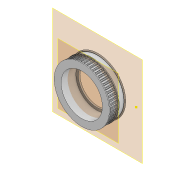
# Autodesk Inventor part: 20_Cube_Insert_rotational_filtermount_v3
Saved by Autodesk Inventor 2022 (Build 260153000, 153)
## iProperties
Created: 2022-02-14
Part Number: 20_Cube_Insert_rotational_filtermount_v3
Material: Generisch
Document SubType Name: Modeling
Designer: diederichbenedict
Density: 1 g/cm^3
Appearance: Vorgabe
Author: diederichbenedict
Autodesk Inventor part; units mm, degrees
ref_plane "YZ Plane" through (0, 0, 0) normal (1, 0, 0) x (0, 1, 0)
ref_plane "XZ Plane" through (0, 0, 0) normal (0, 1, 0) x (-1, 0, 0)
ref_plane "XY Plane" through (0, 0, 0) normal (0, 0, 1) x (1, 0, 0)
ref_plane "Arbeitsebene1" through (0, 0, 0) normal (0, 0, 1) x (1, 0, 0)
sketch "Skizze1" plane through (0, 0, 0) normal (0, 0, 1) x (1, 0, 0)
  circle A0 centre (-23.0919, -0.0207) radius 10 construction
  circle A1 centre (-5.7714, -10.0207) radius 3 construction
  circle A2 centre (-40.4124, -10.0207) radius 3 construction
  circle A3 centre (-23.0919, 19.9793) radius 3 construction
  circle A4 centre (-23.0919, -0.0207) radius 10 construction
  line L0 (1.8288, -17) -> (1.8288, 17) construction
  line L1 (1.8288, 17) -> (-1.746, 17) construction
  line L2 (-1.746, 17) -> (-6.0712, 21.3252) construction
  line L3 (-6.0712, 21.3252) -> (-6.0712, 24.9) construction
  line L4 (-6.0712, 24.9) -> (-40.0712, 24.9) construction
  line L5 (-40.0712, 24.9) -> (-40.0712, 21.3252) construction
  line L6 (-40.0712, 21.3252) -> (-44.3964, 17) construction
  line L7 (-44.3964, 17) -> (-47.9712, 17) construction
  line L8 (-47.9712, 17) -> (-47.9712, -17) construction
  line L9 (-44.3964, -17) -> (-47.9712, -17) construction
  line L10 (-40.0712, -21.3252) -> (-44.3964, -17) construction
  line L11 (-40.0712, -24.9) -> (-40.0712, -21.3252) construction
  line L12 (-6.1126, -24.9) -> (-40.0712, -24.9) construction
  line L13 (-6.1126, -24.9) -> (-6.1126, -21.3666) construction
  line L14 (-6.1126, -21.3666) -> (-1.746, -17) construction
  line L15 (-1.746, -17) -> (1.8288, -17) construction
  circle A5 centre (-23.0919, 19.9793) radius 2.5 construction
  circle A6 centre (-40.4124, -10.0207) radius 2.5 construction
  circle A7 centre (-5.7714, -10.0207) radius 2.5 construction
  circle A8 centre (-23.0919, -0.0207) radius 16.1
  circle A9 centre (-23.0919, 19.9793) radius 4 construction
  circle A10 centre (-5.7714, -10.0207) radius 4 construction
  circle A11 centre (-40.4124, -10.0207) radius 4 construction
  circle A12 centre (-23.0919, -0.0207) radius 12.575
  point P0 (0, 0)
  dimension "d4" = 8
  dimension "d5" = 8
  dimension "d6" = 8
  dimension "d7" = 32.2
  dimension "d8" = 25.15
  constraints: 5 centre point, 4 coincident
  measures "d4" diameter of A9
  measures "d5" diameter of A10
  measures "d6" diameter of A11
  measures "d7" diameter of A8
  measures "d8" diameter of A12
extrude "Extrusion1" add sketch "Skizze1" along normal blind 9
sketch "Skizze2" plane through (-23.0919, -0.0207, 9) normal (0, 0, 1) x (1, 0, 0)
  circle A0 centre (0, 0) radius 16.1 projected
  circle A1 centre (0, 0) radius 12.575 projected
  line L0 (16.6, 0.4) -> (15.6, 0.4)
  line L1 (15.6, 0.4) -> (15.6, -0.4)
  line L2 (15.6, -0.4) -> (16.6, -0.4)
  line L3 (16.6, -0.4) -> (16.6, 0.4)
  circle A2 centre (0, 0) radius 16.1 projected
  line L4 (16.6, 0.4) -> (15.6, -0.4) construction
  line L5 (15.6, 0.4) -> (16.6, -0.4) construction
  point P0 (23.0919, 0.0207)
  point P1 (16.1, 0)
  dimension "d9" = 1
  dimension "d10" = 0.8
  constraints: 12 end point, 2 midpoint, 2 parallel, 1 horizontal, 1 horizontal alignment, 1 perpendicular, 1 other
  measures "d9" distance of L2.end L1.end
  measures "d10" distance of L1.end L0.end
extrude "Extrusion2" add sketch "Skizze2" against normal blind 5 contours A0 L2 L1 L0 | A0 L0 L3 L2 picked at (15.7667, 0)
fillet "Rundung1" radius 0.2 4 edges at (-6.4919, -0.4207, 6.5) (-6.9969, -0.4207, 6.5) (-6.4919, 0.3793, 6.5) (-6.9969, 0.3793, 6.5)
pattern_circular "Runde Anordnung1" count 52 over 360 about axis through (-23.0919, -0.0207, 0) along (0, 0, 1) of "Rundung1", "Extrusion2"
sketch "Skizze3" plane through (0, 0, 9) normal (0, 0, 1) x (1, 0, 0)
  circle A0 centre (-23.0919, -0.0207) radius 12.575 projected
  circle A1 centre (-23.0919, -0.0207) radius 16.7976
  point P0 (0, 0)
  constraints: 1 centre point
extrude "Extrusion3" add sketch "Skizze3" along normal blind 0.5
ref_plane "Arbeitsebene2" through (-23.0919, -0.0207, 5.5) normal (0, 0, 1) x (1, 0, 0)
sketch "Skizze4" plane through (-23.0919, -0.0207, 4) normal (0, 0, 1) x (1, 0, 0)
  circle A0 centre (0, 0) radius 16.7976 projected
  circle A1 centre (0, 0) radius 12.575 projected
  point P0 (23.0919, 0.0207)
extrude "Extrusion4" add sketch "Skizze4" against normal blind 0.5
sketch "Skizze5" plane through (-23.0919, -0.0207, 0) normal (0, 0, -1) x (-1, 0, 0)
  circle A0 centre (0, 0) radius 16.7976 projected
  circle A1 centre (0, 0) radius 12.575 projected
  point P0 (-23.0919, 0.0207)
extrude "Extrusion5" add sketch "Skizze5" along normal blind 0.5
sketch "Skizze6" plane through (-23.0919, -0.0207, -0.5) normal (0, 0, -1) x (-1, 0, 0)
  point P0 (-23.0919, 0.0207)
sketch "Skizze7" plane through (-23.0919, -0.0207, -0.5) normal (0, 0, 1) x (1, 0, 0)
  circle A0 centre (0, 0) radius 12.575 projected
  circle A1 centre (0, 0) radius 11.075
  point P0 (23.0919, 0.0207)
  dimension "d27" = 1.5
  constraints: 1 centre point
  measures "d27" radial gap between concentric circles of A0 A1
extrude "Extrusion6" add sketch "Skizze7" along normal blind 1
chamfer "Fase2" distance 0.5 angle 45 2 edges at (-6.2942, -0.0207, 0) (-39.1919, -0.0207, 3.5)
